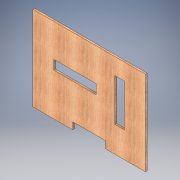
# Autodesk Inventor part: Plywood
Saved by Autodesk Inventor 2018 (Build 220112000, 112)
## iProperties
Created: 2017-09-17
Part Number: Plywood
Material: Generic
Document SubType Name: Modeling
Designer: Techbrick Alt
Density: 1 g/cm^3
Appearance: Birch - Natural Polished
Author: Techbrick Alt
Autodesk Inventor part; units mm, degrees
ref_plane "YZ Plane" through (0, 0, 0) normal (1, 0, 0) x (0, 1, 0)
ref_plane "XZ Plane" through (0, 0, 0) normal (0, 1, 0) x (-1, 0, 0)
ref_plane "XY Plane" through (0, 0, 0) normal (0, 0, 1) x (1, 0, 0)
sketch "Sketch1" plane through (0, 0, 0) normal (0, 0, 1) x (1, 0, 0)
  line L0 (-609.6, 914.4) -> (609.6, 914.4)
  line L1 (609.6, 914.4) -> (609.6, 0)
  line L2 (609.6, 0) -> (-609.6, 0)
  line L3 (-609.6, 0) -> (-609.6, 914.4)
  point P0 (0, 0)
  dimension "d0" = 1219.2
  dimension "d1" = 914.4
  dimension "d2" = 914.4
  dimension "d3" = 609.6
  constraints: 8 end point, 2 parallel, 1 horizontal, 1 perpendicular
  measures "d0" distance of L0.start L0.end
  measures "d1" distance of L2.end L0.start
  measures "d2" distance from line of point (0, 0) L0
  measures "d3" distance from line of point (0, 0) L1
extrude "Plywood" add sketch "Sketch1" along normal blind 19.05
sketch "Sketch2" plane through (0, 0, 19.05) normal (0, 0, 1) x (1, 0, 0)
  line L0 (-177.8, 76.2) -> (177.8, 76.2)
  line L1 (177.8, 76.2) -> (177.8, 0)
  line L2 (177.8, 0) -> (-177.8, 0)
  line L3 (-177.8, 0) -> (-177.8, 76.2)
  line L4 (-609.6, 0) -> (609.6, 0) projected
  line L5 (-381, 558.8) -> (76.2, 558.8)
  line L6 (76.2, 558.8) -> (76.2, 457.2)
  line L7 (76.2, 457.2) -> (-381, 457.2)
  line L8 (-381, 457.2) -> (-381, 558.8)
  line L9 (-381, 508) -> (76.2, 508) construction
  line L10 (279.4, 736.6) -> (381, 736.6)
  line L11 (381, 736.6) -> (381, 279.4)
  line L12 (381, 279.4) -> (279.4, 279.4)
  line L13 (279.4, 279.4) -> (279.4, 736.6)
  line L14 (76.2, 508) -> (279.4, 508)
  point P0 (0, 0)
  dimension "d6" = 355.6
  dimension "d7" = 76.2
  dimension "d8" = 177.8
  dimension "d9" = 457.2
  dimension "d10" = 381
  dimension "d11" = 101.6
  dimension "d12" = 508
  dimension "d15" = 101.6
  dimension "d16" = 457.2
  dimension "d17" = 203.2
  dimension "d18" = 762
  constraints: 28 end point, 6 parallel, 4 horizontal, 3 midpoint, 3 perpendicular, 1 collinear
  measures "d6" distance of L0.start L0.end
  measures "d7" distance of L2.end L0.start
  measures "d8" distance from line of point (0, 0) L1
  measures "d9" distance of L5.start L5.end
  measures "d10" distance from line of point (0, 0) L8
  measures "d11" distance of L5.end L6.end
  measures "d12" distance between parallel lines of L2 L9
  measures "d15" distance of L10.start L10.end
  measures "d16" distance of L10.end L11.end
  measures "d17" distance between parallel lines of L13 L6
  measures "d18" distance between parallel lines of L11 L8
extrude "SLOTS" cut sketch "Sketch2" against normal through all
equation "\"d2\" = d1"
equation "\"d3\" = 0.5 * d0"
equation "\"d8\" = 0.5 * d6"
equation "\"d10\" = 0.5 * d18"
equation "\"d15\" = d11"
equation "\"d16\" = d9"
body "Solid1"
